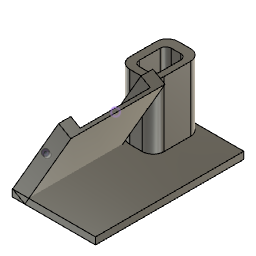
iPhone Doc v1 (Autodesk Fusion 360 design; units mm, degrees)
Autodesk Fusion 360 part; units mm, degrees
sketch "Sketch1" plane through (0, 0, 0) normal (0, 0, 1) x (1, 0, 0)
  line L0 (0, 0) -> (770, 0)
  line L1 (770, 0) -> (770, 1370)
  line L2 (770, 1370) -> (0, 1370)
  line L3 (0, 1370) -> (0, 0)
  dimension "d1" = 770
  dimension "d2" = 1370
  constraint horizontal L0
  constraint vertical L1
  constraint horizontal L2
  constraint vertical L3
  constraint coincident L0.start L3.end
  measures "d1" distance of L0.start L0.end
  measures "d2" distance of L0.start L2.end
extrude "Extrude1" add sketch "Sketch1" along normal blind 64.5 makes body 1
sketch "Sketch2" plane through (0, 0, 0) normal (1, 0, 0) x (0, 1, 0)
  line L0 (0, 65) -> (870, 65)
  line L1 (870, 65) -> (870, 915)
  line L2 (870, 915) -> (0, 915)
  line L3 (0, 915) -> (0, 65)
  point P0 (0, 65)
  point P1 (1368.9003, 64.4486)
  dimension "d5" = 870
  dimension "d6" = 850
  constraint horizontal L0
  constraint vertical L1
  constraint horizontal L2
  constraint vertical L3
  constraint coincident P0 L0.start
  measures "d5" distance of P0 L0.end
  measures "d6" distance of P0 L2.end
extrude "Extrude2" add sketch "Sketch2" along normal blind 130 separate body makes body 2
move_body "Move1" bodies 2 to x (0.866025, 0, -0.5) y (0, 1, 0) z (0.5, 0, 0.866025) at (-27.8311, 0, 9.1241)
sketch "Sketch3" plane through (-24.8242, 0, 14.3322) normal (-0.866025, 0, 0.5) x (0, -1, 0)
  line L0 (0, 58.9862) -> (0, 908.9862)
  line L1 (0, 908.9862) -> (-870, 908.9862)
  line L2 (-870, 908.9862) -> (-870, 58.9862)
  line L3 (-870, 58.9862) -> (0, 58.9862)
  line L4 (-870, 908.9862) -> (-760, 908.9862) construction
  line L5 (0, 908.9862) -> (-110, 908.9862) construction
  line L6 (-760, 908.9862) -> (-760, 588.9862) construction
  line L7 (-760, 908.9862) -> (-112.0008, 908.9862)
  line L8 (-112.0008, 908.9862) -> (-112.0008, 440.6784)
  line L9 (-112.0008, 440.6784) -> (-760, 440.6784)
  line L10 (-760, 440.6784) -> (-760, 908.9862)
  dimension "d9" = 110
  dimension "d10" = 110
  dimension "d11" = 320
  constraint coincident L1.end L2.start
  constraint perpendicular L2 L4
  constraint coincident L0.end L1.start
  constraint perpendicular L0 L5
  constraint perpendicular L4 L6
  constraint horizontal L7
  constraint vertical L8
  constraint horizontal L9
  constraint vertical L10
  measures "d9" distance of L1.end L4.end
  measures "d10" distance of L0.end L5.end
  measures "d11" distance of L4.end L6.end
extrude "Extrude3" cut sketch "Sketch3" against normal blind 100 contours L1 L7 L8 L9 L10 bodies 2
sketch "Sketch4" plane through (220.3392, 0, 381.6387) normal (0.5, 0, 0.866025) x (0, 1, 0)
  line L0 (112.0008, 28.6645) -> (112.0008, -71.3355)
  line L1 (112.0008, -71.3355) -> (760, -71.3355)
  line L2 (760, -71.3355) -> (760, 28.6645)
  line L3 (112.0008, 28.6645) -> (112.0008, 8.6645)
  constraint coincident L0.start L3.start
sketch "Sketch8" plane through (0, 0, 64.5) normal (0, 0, 1) x (-1, 0, 0)
  line L0 (0, -1370) -> (0, 0)
  line L1 (0, 0) -> (-770, 0)
  line L2 (-770, 0) -> (-770, -1370)
  line L3 (-770, -1370) -> (0, -1370)
  line L4 (0, -1370) -> (-385, -1370)
  line L5 (-385, -1370) -> (-385, -866.2848)
  line L6 (-385, -866.2848) -> (0, -866.2848)
  line L7 (0, -866.2848) -> (0, -1370)
  constraint horizontal L4
  constraint vertical L5
  constraint horizontal L6
  constraint vertical L7
  constraint coincident L0.start L3.end
extrude "Extrude8" cut sketch "Sketch8" along normal blind 400 contours L0 L3 L4 L5 L6 L7 bodies 2
sketch "Sketch9" plane through (0, 0, 64.5) normal (0, 0, 1) x (-1, 0, 0)
  line L0 (0, -1370) -> (0, 0)
  line L1 (0, 0) -> (-770, 0)
  line L2 (-770, 0) -> (-770, -1370)
  line L3 (-770, -1370) -> (0, -1370)
  line L4 (-87.36, -1345.2147) -> (-403.9407, -1345.2147)
  line L5 (-403.9407, -1345.2147) -> (-403.9407, -898.7547)
  line L6 (-403.9407, -898.7547) -> (-87.36, -898.7547)
  line L7 (-87.36, -898.7547) -> (-87.36, -1345.2147)
  constraint horizontal L4
  constraint vertical L5
  constraint horizontal L6
  constraint vertical L7
extrude "Extrude9" add sketch "Sketch9" along normal blind 600 contours L4 L5 L6 L7 bodies 1
sketch "Sketch10" plane through (0, 0, 664.5) normal (0, 0, 1) x (-1, 0, 0)
  line L0 (-87.36, -898.7547) -> (-403.9407, -898.7547)
  line L1 (-403.9407, -898.7547) -> (-403.9407, -1345.2147)
  line L2 (-403.9407, -1345.2147) -> (-87.36, -1345.2147)
  line L3 (-87.36, -1345.2147) -> (-87.36, -898.7547)
  line L4 (-159.1256, -1259.5723) -> (-348.5328, -1259.5723)
  line L5 (-348.5328, -1259.5723) -> (-348.5328, -964.6382)
  line L6 (-348.5328, -964.6382) -> (-159.1256, -964.6382)
  line L7 (-159.1256, -964.6382) -> (-159.1256, -1259.5723)
  dimension "d34" = 189.4073
  constraint horizontal L4
  constraint vertical L5
  constraint horizontal L6
  constraint vertical L7
  measures "d34" distance of L4.start L4.end
fillet "Fillet2" radius 100 4 edges at (87.36, 898.7547, 364.5) (87.36, 1345.2147, 364.5) (403.9407, 898.7547, 364.5) (403.9407, 1345.2147, 364.5) on bodies 1
extrude "Extrude10" cut sketch "Sketch10" against normal blind 500 contours L4 L5 L6 L7 bodies 1
fillet "Fillet3" radius 50 4 edges at (159.1256, 964.6382, 414.5) (348.5328, 964.6382, 414.5) (348.5328, 1259.5723, 414.5) (159.1256, 1259.5723, 414.5) on bodies 1
extrude "Extrude4" [suppressed]
sketch "Sketch5" plane through (-24.8242, 0, 14.3322) normal (-0.866025, 0, 0.5) x (0, -1, 0)
  line L0 (-760, 440.6784) -> (-760, 908.9862)
  line L1 (-760, 908.9862) -> (-870, 908.9862)
  line L2 (-870, 908.9862) -> (-870, 58.9862)
  line L3 (-870, 58.9862) -> (0, 58.9862)
  line L4 (0, 58.9862) -> (0, 908.9862)
  line L5 (0, 908.9862) -> (-112.0008, 908.9862)
  line L6 (-112.0008, 908.9862) -> (-112.0008, 440.6784)
  line L7 (-112.0008, 440.6784) -> (-760, 440.6784)
  line L8 (-870, 399.1465) -> (-435, 399.1465) construction
  line L9 (-435, 399.1465) -> (0, 399.1465) construction
  circle A0 centre (-436.0004, 440.6784) radius 69.3907
  point P0 (-435, 399.1465)
  point P1 (-436.0004, 440.6784)
  constraint coincident L2 L8.start
  constraint perpendicular L2 L8
  constraint coincident L4 L9.end
  constraint perpendicular L4 L9
  constraint equal L8 L9
  constraint coincident P0 L8.end
  constraint midpoint L7 P1
  constraint coincident P1 A0.centre
extrude "Extrude5" [suppressed]
sketch "Sketch6" plane through (0, 0, 64.5) normal (0, 0, 1) x (-1, 0, 0)
  line L0 (0, -1370) -> (0, 0)
  line L1 (0, 0) -> (-770, 0)
  line L2 (-770, 0) -> (-770, -1370)
  line L3 (-770, -1370) -> (0, -1370)
  line L4 (0, -850) -> (0, -920)
  dimension "d22" = 70
  constraint coincident L0 L4.start
  constraint parallel L0 L4
  measures "d22" distance of L4.start L4.end
extrude "Extrude6" [suppressed]
sketch "Sketch7" plane through (0, 0, 64.5) normal (0, 0, 1) x (-1, 0, 0)
  line L0 (1.1377, -923.6705) -> (-248.8623, -923.6705)
  line L1 (-248.8623, -923.6705) -> (-248.8623, -1424.2357)
  line L2 (-248.8623, -1424.2357) -> (1.1377, -1424.2357)
  line L3 (1.1377, -1424.2357) -> (1.1377, -923.6705)
  point P0 (1.1377, -923.6705)
  point P1 (1.1377, -1420.1857)
  dimension "d25" = 250
  constraint horizontal L0
  constraint vertical L1
  constraint horizontal L2
  constraint vertical L3
  constraint coincident P0 L0.start
  measures "d25" distance of P0 L0.end
extrude "Extrude7" [suppressed]
fillet "Fillet1" [suppressed]
other "Form1"
moveface "MoveFace2" [suppressed]
shell "Shell1" [suppressed]
